lamp (Autodesk Fusion 360 design; units mm, degrees)
Autodesk Fusion 360 part; units mm, degrees
note: some values were not read from the file. Set by a fixed rule: which sketch regions a step uses.
sketch "Sketch1" plane through (0, 0, 0) normal (0, 1, 0) x (1, 0, 0)
  circle A0 centre (0, 0) radius 19
  circle A1 centre (0, 0) radius 29
  dimension "d1" = 38
  dimension "d2" = 58
  constraint coincident A0.centre A1.centre
  measures "d1" diameter of A0
  measures "d2" diameter of A1
extrude "Extrude1" add sketch "Sketch1" along normal blind 85
thread "Thread1" "ISO Metric profile 42.0 M42x3 6H" major diameter 42.349 minor diameter 39.0024 pitch 3 angle 60 modelled right hand crest width 0.8179 on face at (18.9764, 56.6667, 0.9471) crest through (19.5012, 0.75, 0)
sketch "Sketch2" plane through (0, 0, 0) normal (0, -1, 0) x (1, 0, 0)
  spline S0 degree 3 poles (-5.4799, -20.4531) (-8.0919, -19.6428) (-10.5218, -18.3338) (-14.7064, -14.8784) (-16.4306, -12.7777) (-18.9505, -8.0662) (-19.7357, -5.5085) (-20.2696, -0.2765) (-20.0289, 2.3457) (-18.8496, 6.3305) (-18.2387, 7.758) (-16.7025, 10.4272) (-15.7857, 11.6614) (-14.7337, 12.7755) knots 0 0 0 0 0.820442 0.820442 1.628578 1.628578 2.424403 2.424403 3.207914 3.207914 3.672776 3.672776 4.133133 4.133133 4.133133 4.133133
  arc A0 (14.7337, 12.7755) -> (-14.7337, 12.7755) centre (0, 0) ccw
  spline S1 degree 3 poles (14.7337, 12.7755) (16.4896, 10.9159) (17.8623, 8.7289) (19.7146, 3.915) (20.1615, 1.3289) (20.0457, -3.9116) (19.4683, -6.515) (17.3381, -11.396) (15.7914, -13.6201) (12.6915, -16.6252) (11.3889, -17.6198) (8.5663, -19.2939) (7.0544, -19.9647) (5.4799, -20.4531) knots 0 0 0 0 0.767282 0.767282 1.546861 1.546861 2.338735 2.338735 3.142898 3.142898 3.632202 3.632202 4.126 4.126 4.126 4.126
  arc A1 (-5.4799, -20.4531) -> (5.4799, -20.4531) centre (0, 0) ccw
  circle A2 centre (0, 0) radius 29
  circle A3 centre (0, 0) radius 26
  dimension "d5" = 52
  constraint concentric A0 A3
  measures "d5" diameter of A3
extrude "Extrude2" cut sketch "Sketch2" against normal blind 40 contours S0 A0 S1 A1 | A3
sketch "Sketch3" plane through (0, 0, 0) normal (0, 0, 1) x (1, 0, 0)
  circle A0 centre (0, 4) radius 4
  line L0 (0, -15) -> (0, 39)
  line L1 (-21, 0) -> (23, 0)
  line L2 (-4, 4) -> (4, 4)
  line L3 (4, 4) -> (4, 0)
  line L4 (4, 0) -> (-4, 0)
  line L5 (-4, 0) -> (-4, 4)
  dimension "d8" = 8
  dimension "d9" = 8
  constraint vertical L0
  constraint coincident A0.centre L0
  constraint horizontal L1
  constraint coincident origin A0
  constraint horizontal L2
  constraint vertical L3
  constraint horizontal L4
  constraint vertical L5
  constraint coincident A0.centre L2
  constraint coincident origin L4
  constraint tangent A0 L5
  measures "d8" diameter of A0
  measures "d9" distance of L2.start L2.end
extrude "Extrude3" cut sketch "Sketch3" along normal blind 40
